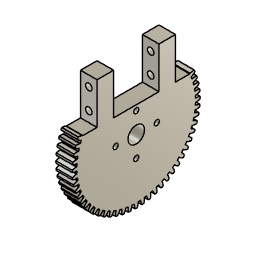
Shaft Arm Joint 0-1 (Autodesk Fusion 360 design; units mm, degrees)
Autodesk Fusion 360 part; units mm, degrees
note: some values were not read from the file. Set by a fixed rule: which sketch regions a step uses.
(part 1 of 59)
sketch "スケッチ1" plane through (0, 0, 0) normal (0, 0, 1) x (1, 0, 0)
  line L0 (4, 19) -> (-4, 19)
  line L1 (-4, 19) -> (-4, -19)
  line L2 (-4, -19) -> (4, -19)
  line L3 (4, -19) -> (4, 19)
  line L4 (4, 19) -> (-4, -19) construction
  line L5 (-4, 19) -> (4, -19) construction
  dimension "d1" = 8
  dimension "d2" = 38
  constraint horizontal L0
  constraint perpendicular L0 L1
  constraint parallel L0 L2
  constraint parallel L1 L3
  constraint coincident L4 origin
  constraint coincident L5 origin
  measures "d1" distance of L1.end L2.end
  measures "d2" distance of L0.end L1.end
extrude "押し出し1" add sketch "スケッチ1" along normal blind 25
sketch "スケッチ4" plane through (4, 0, 0) normal (1, 0, 0) x (0, 1, 0)
  line L0 (-19, 0) -> (19, 0)
  line L1 (19, 0) -> (19, 25)
  line L2 (19, 25) -> (-19, 25)
  line L3 (-19, 25) -> (-19, 0)
  line L4 (0, 25) -> (0, 0)
  circle A0 centre (0, 12.5) radius 12.5
  line L5 (0, 12.5) -> (10, 12.5)
  line L6 (0, 12.5) -> (-10, 12.5)
  line L7 (0, 12.5) -> (0, 22.5)
  line L8 (0, 12.5) -> (0, 2.5)
  line L9 (0, 12.5) -> (7.0711, 5.4289)
  line L10 (0, 12.5) -> (10, 12.5) construction
  line L11 (0, 12.5) -> (7.0711, 19.5711)
  line L12 (0, 12.5) -> (-7.0711, 19.5711)
  line L13 (0, 12.5) -> (-7.0711, 5.4289)
  circle A1 centre (0, 22.5) radius 1.7
  circle A2 centre (7.0711, 19.5711) radius 1.7
  circle A3 centre (10, 12.5) radius 1.7
  circle A4 centre (7.0711, 5.4289) radius 1.7
  circle A5 centre (0, 2.5) radius 1.7
  circle A6 centre (-7.0711, 5.4289) radius 1.7
  circle A7 centre (-10, 12.5) radius 1.7
  circle A8 centre (-7.0711, 19.5711) radius 1.7
  dimension "d11" = 10
  dimension "d12" = 10
  dimension "d13" = 10
  dimension "d14" = 10
  dimension "d15" = 10
  dimension "d16" = 45
  dimension "d17" = 10
  dimension "d18" = 10
  dimension "d19" = 10
  dimension "d20" = 3.4
  dimension "d21" = 3.4
  dimension "d22" = 3.4
  dimension "d23" = 3.4
  dimension "d24" = 3.4
  dimension "d25" = 3.4
  dimension "d26" = 3.4
  dimension "d27" = 3.4
  constraint midpoint L2 L4.start
  constraint coincident L4.end origin
  constraint midpoint L4 A0.centre
  constraint coincident L4.end A0
  constraint coincident A0.centre L5.start
  constraint perpendicular L4 L5
  constraint perpendicular L4 L6
  constraint perpendicular L6 L7
  constraint perpendicular L5 L8
  constraint horizontal L10
  constraint perpendicular L9 L11
  constraint perpendicular L11 L12
  constraint perpendicular L9 L13
  constraint coincident L7.end A1.centre
  constraint coincident L11.end A2.centre
  constraint coincident L5.end L10.end
  constraint coincident L9.end A4.centre
  constraint coincident L8.end A5.centre
  constraint coincident L13.end A6.centre
  constraint coincident L6.end A7.centre
  constraint coincident L12.end A8.centre
  measures "d11" distance of A0.centre L5.end
  measures "d12" distance of A0.centre L6.end
  measures "d13" distance of A0.centre L7.end
  measures "d14" distance of A0.centre L8.end
  measures "d15" distance of A0.centre L9.end
  measures "d16" angle of L9 L10
  measures "d17" distance of A0.centre L11.end
  measures "d18" distance of A0.centre L12.end
  measures "d19" distance of A0.centre L13.end
  measures "d20" diameter of A1
  measures "d21" diameter of A2
  measures "d22" diameter of A3
  measures "d23" diameter of A4
  measures "d24" diameter of A5
  measures "d25" diameter of A6
  measures "d26" diameter of A7
  measures "d27" diameter of A8
extrude "押し出し3" cut sketch "スケッチ4" against normal blind 8 contours L4 L8 A5 | L4 L8 A5 | L4 L7 A1 | L4 L7 A1 | A2 | A3 | A4 | A6 | A7 | A8
sketch "スケッチ6" plane through (0, 0, 25) normal (0, 0, 1) x (-1, 0, 0)
  line L0 (-4, 19) -> (-4, -19)
  line L1 (-4, -19) -> (4, -19)
  line L2 (4, -19) -> (4, 19)
  line L3 (4, 19) -> (-4, 19)
  line L4 (4, -19) -> (-4, -19)
  line L5 (-4, -19) -> (-4, -11)
  line L6 (-4, -11) -> (4, -11)
  line L7 (4, -11) -> (4, -19)
  line L8 (4, 19) -> (-4, 19)
  line L9 (-4, 19) -> (-4, 11)
  line L10 (-4, 11) -> (4, 11)
  line L11 (4, 11) -> (4, 19)
  line L12 (4, -11) -> (-4, -11)
  line L13 (-4, -11) -> (-4, -10)
  line L14 (-4, -10) -> (4, -10)
  line L15 (4, -10) -> (4, -11)
  line L16 (4, 11) -> (-4, 11)
  line L17 (-4, 11) -> (-4, 10)
  line L18 (-4, 10) -> (4, 10)
  line L19 (4, 10) -> (4, 11)
  line L20 (4, -10) -> (-4, -10)
  line L21 (-4, -10) -> (-4, 0)
  line L22 (-4, 0) -> (4, 0)
  line L23 (4, 0) -> (4, -10)
  line L24 (4, 10) -> (-4, 10)
  line L25 (-4, 10) -> (-4, 0)
  line L26 (-4, 0) -> (4, 0)
  line L27 (4, 0) -> (4, 10)
  dimension "d48" = 8
  dimension "d49" = 8
  dimension "d50" = 8
  dimension "d51" = 8
  dimension "d52" = 8
  dimension "d53" = 1
  dimension "d54" = 8
  dimension "d55" = 1
  dimension "d56" = 8
  dimension "d57" = 10
  dimension "d58" = 8
  dimension "d59" = 10
  constraint horizontal L4
  constraint vertical L5
  constraint horizontal L6
  constraint vertical L7
  constraint coincident L1.end L2.start
  constraint horizontal L8
  constraint vertical L9
  constraint horizontal L10
  constraint vertical L11
  constraint coincident L2.end L3.start
  constraint horizontal L12
  constraint vertical L13
  constraint horizontal L14
  constraint vertical L15
  constraint horizontal L16
  constraint vertical L17
  constraint horizontal L18
  constraint vertical L19
  constraint horizontal L20
  constraint vertical L21
  constraint horizontal L22
  constraint vertical L23
  constraint horizontal L24
  constraint vertical L25
  constraint horizontal L26
  constraint vertical L27
  measures "d48" distance of L1.end L0.end
  measures "d49" distance of L1.end L6.end
  measures "d50" distance of L2.end L0.start
  measures "d51" distance of L2.end L10.end
  measures "d52" distance of L6.end L5.end
  measures "d53" distance of L6.end L14.end
  measures "d54" distance of L10.end L9.end
  measures "d55" distance of L10.end L18.end
  measures "d56" distance of L14.end L13.end
  measures "d57" distance of L14.end L22.end
  measures "d58" distance of L18.end L17.end
  measures "d59" distance of L18.end L22.end
extrude "押し出し5" add sketch "スケッチ6" along normal blind 10 contours L0 L2 L3 L8 L9 L10 L11 L16 | L0 L1 L2 L4 L5 L6 L7 L12
sketch "スケッチ7" plane through (4, 0, 0) normal (1, 0, 0) x (0, 1, 0)
  circle A0 centre (-7.0711, 5.4289) radius 1.7
  circle A1 centre (7.0711, 19.5711) radius 1.7
  circle A2 centre (10, 12.5) radius 1.7
  circle A3 centre (0, 2.5) radius 1.7
  circle A4 centre (-10, 12.5) radius 1.7
  circle A5 centre (0, 22.5) radius 1.7
  circle A6 centre (-7.0711, 19.5711) radius 1.7
  circle A7 centre (7.0711, 5.4289) radius 1.7
  line L0 (-19, 0) -> (19, 0)
  line L1 (19, 0) -> (19, 35)
  line L2 (19, 35) -> (11, 35)
  line L3 (11, 35) -> (11, 25)
  line L4 (11, 25) -> (-11, 25)
  line L5 (-11, 25) -> (-11, 35)
  line L6 (-11, 35) -> (-19, 35)
  line L7 (-19, 35) -> (-19, 0)
  circle A8 centre (0, 12.5) radius 12.5
  line L8 (-11, 25) -> (-19, 25)
  line L9 (11, 25) -> (19, 25)
  line L10 (19, 25) -> (11.479, 7.552)
  line L11 (-19, 25) -> (-11.479, 7.552)
  constraint tangent L4 A8
  constraint coincident L4.end L5.start
  constraint coincident L7 L8.end
  constraint perpendicular L7 L8
  constraint coincident L3.end L4.start
  constraint coincident L1 L9.end
  constraint perpendicular L1 L9
  constraint coincident A8 L10.end
  constraint tangent A8 L10
  constraint coincident A8 L11.end
  constraint tangent A8 L11
extrude "押し出し6" cut sketch "スケッチ7" against normal blind 8 contours L0 L7 A8 L11 | L0 L1 A8 L10
sketch "スケッチ8" plane through (4, 0, 0) normal (1, 0, 0) x (0, 1, 0)
  circle A0 centre (7.0711, 5.4289) radius 1.7
  circle A1 centre (-7.0711, 19.5711) radius 1.7
  circle A2 centre (0, 22.5) radius 1.7
  circle A3 centre (-10, 12.5) radius 1.7
  circle A4 centre (0, 2.5) radius 1.7
  circle A5 centre (10, 12.5) radius 1.7
  circle A6 centre (7.0711, 19.5711) radius 1.7
  circle A7 centre (-7.0711, 5.4289) radius 1.7
  line L0 (-19, 25) -> (-11.479, 7.552)
  arc A8 (-11.479, 7.552) -> (11.479, 7.552) centre (0, 12.5) ccw
  line L1 (11.479, 7.552) -> (19, 25)
  line L2 (19, 25) -> (19, 35)
  line L3 (19, 35) -> (11, 35)
  line L4 (11, 35) -> (11, 25)
  line L5 (11, 25) -> (-11, 25)
  line L6 (-11, 25) -> (-11, 35)
  line L7 (-11, 35) -> (-19, 35)
  line L8 (-19, 35) -> (-19, 25)
  circle A9 centre (0, 12.5) radius 13.7
  line L9 (19, 25) -> (12.9047, 7.9001)
  line L10 (-19, 25) -> (-12.9047, 7.9001)
  dimension "d64" = 27.4
  constraint concentric A8 A9
  constraint coincident L1.end L2.start
  constraint coincident A9 L9.end
  constraint tangent A9 L9
  constraint coincident L0.start L8.end
  constraint coincident A9 L10.end
  constraint tangent A9 L10
  measures "d64" diameter of A9
extrude "押し出し7" add sketch "スケッチ8" against normal blind 8 contours L0 A9 L10 | L0 A8 L1 A9 | L1 A9 L9
sketch "スケッチ9" plane through (4, 0, 0) normal (1, 0, 0) x (0, 1, 0)
  circle A0 centre (7.0711, 5.4289) radius 1.7
  circle A1 centre (-7.0711, 19.5711) radius 1.7
  circle A2 centre (0, 22.5) radius 1.7
  circle A3 centre (-10, 12.5) radius 1.7
  circle A4 centre (0, 2.5) radius 1.7
  circle A5 centre (10, 12.5) radius 1.7
  circle A6 centre (7.0711, 19.5711) radius 1.7
  circle A7 centre (-7.0711, 5.4289) radius 1.7
  line L0 (-19, 25) -> (-12.9047, 7.9001)
  arc A8 (-12.9047, 7.9001) -> (12.9047, 7.9001) centre (0, 12.5) ccw
  line L1 (12.9047, 7.9001) -> (19, 25)
  line L2 (19, 25) -> (19, 35)
  line L3 (19, 35) -> (11, 35)
  line L4 (11, 35) -> (11, 25)
  line L5 (11, 25) -> (-11, 25)
  line L6 (-11, 25) -> (-11, 35)
  line L7 (-11, 35) -> (-19, 35)
  line L8 (-19, 35) -> (-19, 25)
  line L9 (0, 12.5) -> (0, 12.2)
  line L10 (0, 12.5) -> (0, 12.8)
  line L11 (3, 12.2) -> (-3, 12.2)
  line L12 (-3, 12.2) -> (-3, 12.8)
  line L13 (-3, 12.8) -> (3, 12.8)
  line L14 (3, 12.8) -> (3, 12.2)
  line L15 (3, 12.2) -> (-3, 12.8) construction
  line L16 (-3, 12.2) -> (3, 12.8) construction
  line L17 (0, 12.8) -> (0, 15.3)
  line L18 (0, 12.2) -> (0, 9.7)
  circle A9 centre (0, 12.8) radius 3
  circle A10 centre (0, 12.2) radius 3
  point P0 (0, 12.5)
  dimension "d69" = 0.3
  dimension "d70" = 0.3
  dimension "d71" = 6
  dimension "d72" = 2.5
  dimension "d73" = 2.5
  constraint coincident P0 A8.centre
  constraint vertical L9
  constraint parallel L9 L10
  constraint horizontal L11
  constraint perpendicular L11 L12
  constraint parallel L11 L13
  constraint parallel L12 L14
  constraint coincident L15 P0
  constraint coincident L16 P0
  constraint perpendicular L13 L17
  constraint perpendicular L11 L18
  constraint coincident L10.end L17.start
  constraint coincident L13.end A9
  constraint coincident L11.start A10
  measures "d69" distance of P0 L9.end
  measures "d70" distance of P0 L10.end
  measures "d71" distance of L12.end L13.end
  measures "d72" distance of L10.end L17.end
  measures "d73" distance of L9.end L18.end
extrude "押し出し8" cut sketch "スケッチ9" against normal blind 8 contours L11 L18 A9 | L11 L18 A9 | L13 L17 A10 | L13 L17 A10 | L11 A9 A10 | L13 A9 A10 picked at (0, 9.4056) picked at (0, 15.5944)
sketch "スケッチ10" plane through (4, 0, 0) normal (1, 0, 0) x (0, 1, 0)
  line L0 (3, 12.8) -> (-3, 12.8)
  arc A0 (3, 12.8) -> (-3, 12.8) centre (0, 12.8) ccw
  arc A1 (-3, 12.2) -> (3, 12.2) centre (0, 12.2) ccw
  line L1 (-3, 12.2) -> (3, 12.2)
  circle A2 centre (7.0711, 5.4289) radius 1.7
  circle A3 centre (-7.0711, 19.5711) radius 1.7
  circle A4 centre (0, 22.5) radius 1.7
  circle A5 centre (-10, 12.5) radius 1.7
  circle A6 centre (0, 2.5) radius 1.7
  circle A7 centre (10, 12.5) radius 1.7
  circle A8 centre (7.0711, 19.5711) radius 1.7
  circle A9 centre (-7.0711, 5.4289) radius 1.7
  line L2 (-19, 25) -> (-12.9047, 7.9001)
  arc A10 (-12.9047, 7.9001) -> (12.9047, 7.9001) centre (0, 12.5) ccw
  line L3 (12.9047, 7.9001) -> (19, 25)
  line L4 (19, 25) -> (19, 35)
  line L5 (19, 35) -> (11, 35)
  line L6 (11, 35) -> (11, 25)
  line L7 (11, 25) -> (-11, 25)
  line L8 (-11, 25) -> (-11, 35)
  line L9 (-11, 35) -> (-19, 35)
  line L10 (-19, 35) -> (-19, 25)
  line L11 (-19, 25) -> (-20, 25)
  line L12 (19, 25) -> (20, 25)
  line L13 (-20, 25) -> (-12.6588, 7.2612)
  line L14 (20, 25) -> (12.6588, 7.2612)
  dimension "d76" = 1
  dimension "d77" = 1
  constraint coincident L2.start L10.end
  constraint perpendicular L10 L11
  constraint coincident L3.end L4.start
  constraint perpendicular L4 L12
  constraint coincident A10 L13.end
  constraint tangent A10 L13
  constraint coincident A10 L14.end
  constraint tangent A10 L14
  measures "d76" distance of L2.start L11.end
  measures "d77" distance of L3.end L12.end
extrude "押し出し9" add sketch "スケッチ10" against normal blind 8 contours L2 A10 L11 L13 | A10 L3 L12 L14
cylinder "円柱プリミティブ1" cut diameter 3.4 height -38 placed x (1, 0, 0) y (0, 0, 1) z (0, -1, 0) at (0, -19, 30)
sketch "スケッチ15" plane through (4, 0, 0) normal (1, 0, 0) x (0, 1, 0)
  line L0 (3, 12.8) -> (-3, 12.8)
  arc A0 (3, 12.8) -> (-3, 12.8) centre (0, 12.8) ccw
  arc A1 (-3, 12.2) -> (3, 12.2) centre (0, 12.2) ccw
  line L1 (-3, 12.2) -> (3, 12.2)
  circle A2 centre (7.0711, 5.4289) radius 1.7
  circle A3 centre (-7.0711, 19.5711) radius 1.7
  circle A4 centre (0, 22.5) radius 1.7
  circle A5 centre (-10, 12.5) radius 1.7
  circle A6 centre (0, 2.5) radius 1.7
  circle A7 centre (10, 12.5) radius 1.7
  circle A8 centre (7.0711, 19.5711) radius 1.7
  circle A9 centre (-7.0711, 5.4289) radius 1.7
  arc A10 (-12.6588, 7.2612) -> (12.6588, 7.2612) centre (0, 12.5) ccw
  line L2 (12.6588, 7.2612) -> (20, 25)
  line L3 (20, 25) -> (19, 25)
  line L4 (19, 25) -> (19, 35)
  line L5 (19, 35) -> (11, 35)
  line L6 (11, 35) -> (11, 25)
  line L7 (11, 25) -> (-11, 25)
  line L8 (-11, 25) -> (-11, 35)
  line L9 (-11, 35) -> (-19, 35)
  line L10 (-19, 35) -> (-19, 25)
  line L11 (-19, 25) -> (-20, 25)
  line L12 (-20, 25) -> (-12.6588, 7.2612)
  line L13 (22.1904, -6.2406) -> (22.1898, -6.2401)
  line L14 (26.6221, 23.3547) -> (26.8948, 23.4659)
  line L15 (25.3417, 26.078) -> (25.6012, 26.2171)
  line L16 (17.8091, -10.4448) -> (17.8086, -10.4441)
  line L17 (17.8086, -10.4441) -> (17.6281, -10.2115)
  spline S0 degree 5 poles (27.8945, 20.5948) (27.8946, 20.5948) (27.8948, 20.5948) (27.8951, 20.5949) (27.8956, 20.5951) (27.8963, 20.5953) (27.8971, 20.5956) (27.898, 20.5958) (27.8991, 20.5962) (27.9002, 20.5965) (27.9015, 20.5969) (27.9028, 20.5973) (27.9043, 20.5978) (27.9058, 20.5983) (27.9075, 20.5988) (27.9092, 20.5994) (27.9111, 20.6) (27.913, 20.6007) (27.915, 20.6013) (27.9172, 20.602) (27.9194, 20.6028) (27.9217, 20.6036) (27.9241, 20.6044) (27.9265, 20.6052) (27.9291, 20.6061) (27.9318, 20.607) (27.9345, 20.608) (27.9373, 20.609) (27.9402, 20.61) (27.9432, 20.6111) (27.9462, 20.6121) (27.9494, 20.6133) (27.9526, 20.6144) (27.9559, 20.6156) (27.9593, 20.6169) (27.9627, 20.6181) (27.9662, 20.6194) (27.9698, 20.6208) (27.9735, 20.6222) (27.9772, 20.6236) (27.9811, 20.625) (27.9849, 20.6265) (27.9889, 20.628) (27.9929, 20.6295) (27.997, 20.6311) (28.0012, 20.6327) (28.0054, 20.6344) (28.0097, 20.6361) (28.0141, 20.6378) (28.0185, 20.6395) (28.023, 20.6413) (28.0276, 20.6432) (28.0322, 20.645) (28.0369, 20.6469) (28.0416, 20.6488) (28.0464, 20.6508) (28.0513, 20.6528) (28.0562, 20.6548) (28.0612, 20.6569) (28.0663, 20.659) (28.0714, 20.6611) (28.0765, 20.6633) (28.0818, 20.6655) (28.087, 20.6677) (28.0924, 20.67) (28.0978, 20.6723) (28.1032, 20.6747) (28.1087, 20.677) (28.1143, 20.6795) (28.1199, 20.6819) (28.1256, 20.6844) (28.1313, 20.6869) (28.1371, 20.6895) (28.1429, 20.692) (28.1488, 20.6947) (28.1547, 20.6973) (28.1607, 20.7) (28.1667, 20.7027) (28.1728, 20.7055) (28.179, 20.7083) (28.1851, 20.7111) (28.1914, 20.714) (28.1977, 20.7169) (28.204, 20.7198) (28.2104, 20.7227) (28.2168, 20.7257) (28.2233, 20.7288) (28.2298, 20.7318) (28.2363, 20.7349) (28.2429, 20.7381) (28.2496, 20.7412) (28.2563, 20.7445) (28.263, 20.7477) (28.2698, 20.751) (28.2767, 20.7543) (28.2835, 20.7576) (28.2905, 20.761) (28.2974, 20.7644) (28.3044, 20.7678) (28.3115, 20.7713) (28.3186, 20.7748) (28.3257, 20.7784) (28.3329, 20.782) (28.3401, 20.7856) (28.3473, 20.7892) (28.3546, 20.7929) (28.3619, 20.7966) (28.3693, 20.8004) (28.3767, 20.8042) (28.3842, 20.808) (28.3917, 20.8118) (28.3992, 20.8157) (28.4068, 20.8196) (28.4144, 20.8236) (28.422, 20.8276) (28.4297, 20.8316) (28.4374, 20.8357) (28.4452, 20.8398) (28.4529, 20.8439) (28.4608, 20.848) (28.4686, 20.8522) (28.4765, 20.8565) (28.4845, 20.8607) (28.4924, 20.865) (28.5004, 20.8693) (28.5085, 20.8737) (28.5165, 20.8781) (28.5246, 20.8825) (28.5328, 20.887) (28.5409, 20.8915) (28.5491, 20.896) (28.5574, 20.9006) (28.5657, 20.9052) (28.574, 20.9098) (28.5823, 20.9145) (28.5907, 20.9192) (28.5991, 20.9239) (28.6075, 20.9287) (28.616, 20.9335) (28.6244, 20.9384) (28.633, 20.9432) (28.6415, 20.9481) (28.6501, 20.9531) (28.6587, 20.958) (28.6674, 20.963) (28.676, 20.9681) (28.6847, 20.9732) (28.6935, 20.9783) (28.7022, 20.9834) (28.711, 20.9886) (28.7199, 20.9938) (28.7287, 20.999) (28.7376, 21.0043) (28.7465, 21.0096) (28.7554, 21.015) (28.7644, 21.0203) (28.7734, 21.0257) (28.7824, 21.0312) (28.7914, 21.0367) (28.8005, 21.0422) (28.8096, 21.0477) (28.8187, 21.0533) (28.8279, 21.0589) (28.837, 21.0645) (28.8462, 21.0702) (28.8555, 21.0759) (28.8647, 21.0817) (28.874, 21.0874) (28.8833, 21.0932) (28.8926, 21.0991) (28.902, 21.105) (28.9113, 21.1109) (28.9207, 21.1168) (28.9302, 21.1228) (28.9396, 21.1288) (28.9491, 21.1348) (28.9586, 21.1409) (28.9681, 21.147) (28.9776, 21.1532) (28.9872, 21.1593) (28.9968, 21.1656) (29.0064, 21.1718) (29.016, 21.1781) (29.0257, 21.1844) (29.0354, 21.1907) (29.0451, 21.1971) (29.0548, 21.2035) (29.0646, 21.2099) (29.0743, 21.2164) (29.0841, 21.2229) (29.0939, 21.2295) (29.1037, 21.236) (29.1136, 21.2426) (29.1235, 21.2493) (29.1334, 21.2559) (29.1433, 21.2626) (29.1532, 21.2694) (29.1632, 21.2762) (29.1731, 21.283) (29.1831, 21.2898) (29.1932, 21.2967) (29.2032, 21.3036) (29.2132, 21.3105) (29.2233, 21.3175) (29.2334, 21.3245) (29.2435, 21.3315) (29.2537, 21.3386) (29.2638, 21.3457) (29.274, 21.3528) (29.2842, 21.36) (29.2944, 21.3671) (29.3046, 21.3744) (29.3148, 21.3816) (29.3251, 21.3889) (29.3354, 21.3963) (29.3457, 21.4036) (29.356, 21.411) (29.3663, 21.4184) (29.3766, 21.4259) (29.387, 21.4334) (29.3974, 21.4409) (29.4078, 21.4485) (29.4182, 21.456) (29.4286, 21.4637) (29.4391, 21.4713) (29.4495, 21.479) (29.46, 21.4867) (29.4705, 21.4945) (29.481, 21.5022) (29.4915, 21.5101) (29.5021, 21.5179) (29.5127, 21.5258) (29.5232, 21.5337) (29.5338, 21.5416) (29.5444, 21.5496) (29.555, 21.5576) (29.5657, 21.5657) (29.5763, 21.5737) (29.587, 21.5818) (29.5977, 21.59) (29.6084, 21.5981) (29.6169, 21.6047) (29.6234, 21.6096) (29.6276, 21.6129) (29.6298, 21.6146) knots 0 0 0 0 0 0 0.00416667 0.00833333 0.0125 0.01666667 0.02083333 0.025 0.02916667 0.03333333 0.0375 0.04166667 0.04583333 0.05 0.05416667 0.05833333 0.0625 0.06666667 0.07083333 0.075 0.07916667 0.08333333 0.0875 0.09166667 0.09583333 0.1 0.10416667 0.10833333 0.1125 0.11666667 0.12083333 0.125 0.12916667 0.13333333 0.1375 0.14166667 0.14583333 0.15 0.15416667 0.15833333 0.1625 0.16666667 0.17083333 0.175 0.17916667 0.18333333 0.1875 0.19166667 0.19583333 0.2 0.20416667 0.20833333 0.2125 0.21666667 0.22083333 0.225 0.22916667 0.23333333 0.2375 0.24166667 0.24583333 0.25 0.25416667 0.25833333 0.2625 0.26666667 0.27083333 0.275 0.27916667 0.28333333 0.2875 0.29166667 0.29583333 0.3 0.30416667 0.30833333 0.3125 0.31666667 0.32083333 0.325 0.32916667 0.33333333 0.3375 0.34166667 0.34583333 0.35 0.35416667 0.35833333 0.3625 0.36666667 0.37083333 0.375 0.37916667 0.38333333 0.3875 0.39166667 0.39583333 0.4 0.40416667 0.40833333 0.4125 0.41666667 0.42083333 0.425 0.42916667 0.43333333 0.4375 0.44166667 0.44583333 0.45 0.45416667 0.45833333 0.4625 0.46666667 0.47083333 0.475 0.47916667 0.48333333 0.4875 0.49166667 0.49583333 0.5 0.50416667 0.50833333 0.5125 0.51666667 0.52083333 0.525 0.52916667 0.53333333 0.5375 0.54166667 0.54583333 0.55 0.55416667 0.55833333 0.5625 0.56666667 0.57083333 0.575 0.57916667 0.58333333 0.5875 0.59166667 0.59583333 0.6 0.60416667 0.60833333 0.6125 0.61666667 0.62083333 0.625 0.62916667 0.63333333 0.6375 0.64166667 0.64583333 0.65 0.65416667 0.65833333 0.6625 0.66666667 0.67083333 0.675 0.67916667 0.68333333 0.6875 0.69166667 0.69583333 0.7 0.70416667 0.70833333 0.7125 0.71666667 0.72083333 0.725 0.72916667 0.73333333 0.7375 0.74166667 0.74583333 0.75 0.75416667 0.75833333 0.7625 0.76666667 0.77083333 0.775 0.77916667 0.78333333 0.7875 0.79166667 0.79583333 0.8 0.80416667 0.80833333 0.8125 0.81666667 0.82083333 0.825 0.82916667 0.83333333 0.8375 0.84166667 0.84583333 0.85 0.85416667 0.85833333 0.8625 0.86666667 0.87083333 0.875 0.87916667 0.88333333 0.8875 0.89166667 0.89583333 0.9 0.90416667 0.90833333 0.9125 0.91666667 0.92083333 0.925 0.92916667 0.93333333 0.9375 0.94166667 0.94583333 0.95 0.95416667 0.95833333 0.9625 0.96666667 0.97083333 0.975 0.97916667 0.98333333 0.9875 0.99166667 0.99583333 1 1 1 1 1 1
  spline S1 degree 5 poles (3.7249, -18.2754) (3.7256, -18.2728) (3.7268, -18.2675) (3.7287, -18.2596) (3.7312, -18.2491) (3.7343, -18.236) (3.7374, -18.223) (3.7405, -18.2099) (3.7435, -18.1969) (3.7466, -18.1839) (3.7496, -18.171) (3.7525, -18.158) (3.7555, -18.1451) (3.7584, -18.1323) (3.7613, -18.1194) (3.7642, -18.1066) (3.767, -18.0938) (3.7699, -18.081) (3.7727, -18.0683) (3.7755, -18.0556) (3.7782, -18.0429) (3.781, -18.0302) (3.7837, -18.0176) (3.7864, -18.005) (3.7891, -17.9924) (3.7917, -17.9799) (3.7943, -17.9674) (3.797, -17.9549) (3.7995, -17.9424) (3.8021, -17.93) (3.8046, -17.9176) (3.8071, -17.9053) (3.8096, -17.8929) (3.8121, -17.8806) (3.8145, -17.8683) (3.817, -17.8561) (3.8194, -17.8439) (3.8217, -17.8317) (3.8241, -17.8195) (3.8264, -17.8074) (3.8288, -17.7953) (3.831, -17.7832) (3.8333, -17.7712) (3.8356, -17.7592) (3.8378, -17.7472) (3.84, -17.7353) (3.8422, -17.7233) (3.8443, -17.7115) (3.8464, -17.6996) (3.8486, -17.6878) (3.8507, -17.676) (3.8527, -17.6643) (3.8548, -17.6525) (3.8568, -17.6409) (3.8588, -17.6292) (3.8608, -17.6176) (3.8628, -17.606) (3.8647, -17.5944) (3.8666, -17.5829) (3.8685, -17.5714) (3.8704, -17.56) (3.8722, -17.5486) (3.8741, -17.5372) (3.8759, -17.5258) (3.8777, -17.5145) (3.8795, -17.5032) (3.8812, -17.492) (3.8829, -17.4807) (3.8846, -17.4696) (3.8863, -17.4584) (3.888, -17.4473) (3.8896, -17.4362) (3.8913, -17.4252) (3.8929, -17.4142) (3.8945, -17.4032) (3.896, -17.3923) (3.8976, -17.3814) (3.8991, -17.3705) (3.9006, -17.3597) (3.9021, -17.3489) (3.9035, -17.3382) (3.905, -17.3274) (3.9064, -17.3168) (3.9078, -17.3061) (3.9092, -17.2955) (3.9106, -17.285) (3.9119, -17.2744) (3.9132, -17.264) (3.9145, -17.2535) (3.9158, -17.2431) (3.9171, -17.2327) (3.9183, -17.2224) (3.9196, -17.2121) (3.9208, -17.2018) (3.922, -17.1916) (3.9231, -17.1814) (3.9243, -17.1713) (3.9254, -17.1612) (3.9265, -17.1512) (3.9276, -17.1411) (3.9287, -17.1312) (3.9297, -17.1212) (3.9308, -17.1113) (3.9318, -17.1015) (3.9328, -17.0917) (3.9338, -17.0819) (3.9348, -17.0722) (3.9357, -17.0625) (3.9366, -17.0529) (3.9375, -17.0433) (3.9384, -17.0337) (3.9393, -17.0242) (3.9402, -17.0147) (3.941, -17.0053) (3.9418, -16.9959) (3.9426, -16.9866) (3.9434, -16.9773) (3.9442, -16.968) (3.9449, -16.9588) (3.9457, -16.9497) (3.9464, -16.9406) (3.9471, -16.9315) (3.9478, -16.9225) (3.9484, -16.9135) (3.9491, -16.9045) (3.9497, -16.8957) (3.9503, -16.8868) (3.9509, -16.878) (3.9515, -16.8693) (3.9521, -16.8606) (3.9526, -16.8519) (3.9532, -16.8433) (3.9537, -16.8348) (3.9542, -16.8263) (3.9547, -16.8178) (3.9552, -16.8094) (3.9556, -16.801) (3.9561, -16.7927) (3.9565, -16.7845) (3.9569, -16.7763) (3.9573, -16.7681) (3.9577, -16.76) (3.9581, -16.7519) (3.9584, -16.7439) (3.9588, -16.736) (3.9591, -16.7281) (3.9594, -16.7202) (3.9597, -16.7124) (3.96, -16.7047) (3.9603, -16.697) (3.9605, -16.6893) (3.9607, -16.6817) (3.961, -16.6742) (3.9612, -16.6667) (3.9614, -16.6593) (3.9616, -16.6519) (3.9618, -16.6446) (3.9619, -16.6374) (3.9621, -16.6302) (3.9622, -16.623) (3.9623, -16.6159) (3.9625, -16.6089) (3.9626, -16.6019) (3.9626, -16.595) (3.9627, -16.5882) (3.9628, -16.5814) (3.9628, -16.5746) (3.9629, -16.568) (3.9629, -16.5613) (3.9629, -16.5548) (3.963, -16.5483) (3.963, -16.5418) (3.9629, -16.5355) (3.9629, -16.5291) (3.9629, -16.5229) (3.9629, -16.5167) (3.9628, -16.5106) (3.9627, -16.5045) (3.9627, -16.4985) (3.9626, -16.4926) (3.9625, -16.4867) (3.9624, -16.4809) (3.9623, -16.4752) (3.9622, -16.4695) (3.9621, -16.4639) (3.962, -16.4584) (3.9618, -16.4529) (3.9617, -16.4475) (3.9615, -16.4422) (3.9614, -16.4369) (3.9612, -16.4317) (3.961, -16.4266) (3.9609, -16.4215) (3.9607, -16.4166) (3.9605, -16.4117) (3.9603, -16.4068) (3.9601, -16.4021) (3.9599, -16.3974) (3.9597, -16.3928) (3.9595, -16.3882) (3.9593, -16.3838) (3.959, -16.3794) (3.9588, -16.3751) (3.9586, -16.3709) (3.9584, -16.3667) (3.9581, -16.3626) (3.9579, -16.3586) (3.9577, -16.3547) (3.9574, -16.3509) (3.9572, -16.3472) (3.9569, -16.3435) (3.9567, -16.3399) (3.9564, -16.3364) (3.9562, -16.333) (3.9559, -16.3297) (3.9557, -16.3264) (3.9555, -16.3233) (3.9552, -16.3202) (3.955, -16.3172) (3.9547, -16.3144) (3.9545, -16.3116) (3.9543, -16.3089) (3.954, -16.3063) (3.9538, -16.3037) (3.9536, -16.3013) (3.9534, -16.299) (3.9531, -16.2968) (3.9529, -16.2946) (3.9527, -16.2926) (3.9525, -16.2907) (3.9523, -16.2889) (3.9522, -16.2871) (3.952, -16.2855) (3.9518, -16.284) (3.9517, -16.2826) (3.9515, -16.2813) (3.9514, -16.2801) (3.9512, -16.279) (3.9511, -16.278) (3.951, -16.2772) (3.9509, -16.2764) (3.9509, -16.2759) (3.9508, -16.2756) (3.9508, -16.2754) (3.9508, -16.2753) knots -1 -1 -1 -1 -1 -1 -0.99583333 -0.99166667 -0.9875 -0.98333333 -0.97916667 -0.975 -0.97083333 -0.96666667 -0.9625 -0.95833333 -0.95416667 -0.95 -0.94583333 -0.94166667 -0.9375 -0.93333333 -0.92916667 -0.925 -0.92083333 -0.91666667 -0.9125 -0.90833333 -0.90416667 -0.9 -0.89583333 -0.89166667 -0.8875 -0.88333333 -0.87916667 -0.875 -0.87083333 -0.86666667 -0.8625 -0.85833333 -0.85416667 -0.85 -0.84583333 -0.84166667 -0.8375 -0.83333333 -0.82916667 -0.825 -0.82083333 -0.81666667 -0.8125 -0.80833333 -0.80416667 -0.8 -0.79583333 -0.79166667 -0.7875 -0.78333333 -0.77916667 -0.775 -0.77083333 -0.76666667 -0.7625 -0.75833333 -0.75416667 -0.75 -0.74583333 -0.74166667 -0.7375 -0.73333333 -0.72916667 -0.725 -0.72083333 -0.71666667 -0.7125 -0.70833333 -0.70416667 -0.7 -0.69583333 -0.69166667 -0.6875 -0.68333333 -0.67916667 -0.675 -0.67083333 -0.66666667 -0.6625 -0.65833333 -0.65416667 -0.65 -0.64583333 -0.64166667 -0.6375 -0.63333333 -0.62916667 -0.625 -0.62083333 -0.61666667 -0.6125 -0.60833333 -0.60416667 -0.6 -0.59583333 -0.59166667 -0.5875 -0.58333333 -0.57916667 -0.575 -0.57083333 -0.56666667 -0.5625 -0.55833333 -0.55416667 -0.55 -0.54583333 -0.54166667 -0.5375 -0.53333333 -0.52916667 -0.525 -0.52083333 -0.51666667 -0.5125 -0.50833333 -0.50416667 -0.5 -0.49583333 -0.49166667 -0.4875 -0.48333333 -0.47916667 -0.475 -0.47083333 -0.46666667 -0.4625 -0.45833333 -0.45416667 -0.45 -0.44583333 -0.44166667 -0.4375 -0.43333333 -0.42916667 -0.425 -0.42083333 -0.41666667 -0.4125 -0.40833333 -0.40416667 -0.4 -0.39583333 -0.39166667 -0.3875 -0.38333333 -0.37916667 -0.375 -0.37083333 -0.36666667 -0.3625 -0.35833333 -0.35416667 -0.35 -0.34583333 -0.34166667 -0.3375 -0.33333333 -0.32916667 -0.325 -0.32083333 -0.31666667 -0.3125 -0.30833333 -0.30416667 -0.3 -0.29583333 -0.29166667 -0.2875 -0.28333333 -0.27916667 -0.275 -0.27083333 -0.26666667 -0.2625 -0.25833333 -0.25416667 -0.25 -0.24583333 -0.24166667 -0.2375 -0.23333333 -0.22916667 -0.225 -0.22083333 -0.21666667 -0.2125 -0.20833333 -0.20416667 -0.2 -0.19583333 -0.19166667 -0.1875 -0.18333333 -0.17916667 -0.175 -0.17083333 -0.16666667 -0.1625 -0.15833333 -0.15416667 -0.15 -0.14583333 -0.14166667 -0.1375 -0.13333333 -0.12916667 -0.125 -0.12083333 -0.11666667 -0.1125 -0.10833333 -0.10416667 -0.1 -0.09583333 -0.09166667 -0.0875 -0.08333333 -0.07916667 -0.075 -0.07083333 -0.06666667 -0.0625 -0.05833333 -0.05416667 -0.05 -0.04583333 -0.04166667 -0.0375 -0.03333333 -0.02916667 -0.025 -0.02083333 -0.01666667 -0.0125 -0.00833333 -0.00416667 0 0 0 0 0 0
  line L18 (24.6799, 27.8128) -> (24.4297, 27.6575)
  arc A11 (29.6298, 21.6146) -> (29.3284, 22.5421) centre (0, 12.5) ccw
  line L19 (26.8948, 23.4659) -> (26.8955, 23.4662)
  line L20 (24.0278, -3.8184) -> (24.0271, -3.818)
  line L21 (24.0271, -3.818) -> (23.7836, -3.6526)
  line L22 (24.6806, 27.8132) -> (24.6799, 27.8128)
  arc A12 (30.4202, 18.4675) -> (30.2174, 19.4214) centre (0, 12.5) ccw
  arc A13 (27.918, 19.3665) -> (27.6109, 20.5125) centre (0, 12.5) ccw
  spline S2 degree 5 poles (-5.9675, -17.9202) (-5.9661, -17.9179) (-5.9633, -17.9133) (-5.959, -17.9064) (-5.9534, -17.8972) (-5.9464, -17.8857) (-5.9394, -17.8742) (-5.9325, -17.8628) (-5.9255, -17.8513) (-5.9187, -17.8399) (-5.9118, -17.8285) (-5.905, -17.8171) (-5.8982, -17.8058) (-5.8914, -17.7944) (-5.8847, -17.7831) (-5.878, -17.7718) (-5.8713, -17.7605) (-5.8647, -17.7492) (-5.8581, -17.738) (-5.8515, -17.7268) (-5.8449, -17.7156) (-5.8384, -17.7044) (-5.8319, -17.6932) (-5.8255, -17.6821) (-5.8191, -17.6709) (-5.8127, -17.6598) (-5.8063, -17.6487) (-5.8, -17.6377) (-5.7937, -17.6266) (-5.7874, -17.6156) (-5.7811, -17.6046) (-5.7749, -17.5936) (-5.7688, -17.5826) (-5.7626, -17.5717) (-5.7565, -17.5608) (-5.7504, -17.5499) (-5.7443, -17.539) (-5.7383, -17.5281) (-5.7323, -17.5173) (-5.7263, -17.5065) (-5.7204, -17.4957) (-5.7145, -17.4849) (-5.7086, -17.4742) (-5.7028, -17.4634) (-5.697, -17.4527) (-5.6912, -17.4421) (-5.6854, -17.4314) (-5.6797, -17.4208) (-5.674, -17.4102) (-5.6683, -17.3996) (-5.6627, -17.389) (-5.6571, -17.3785) (-5.6515, -17.368) (-5.646, -17.3575) (-5.6405, -17.347) (-5.635, -17.3366) (-5.6296, -17.3262) (-5.6242, -17.3158) (-5.6188, -17.3054) (-5.6134, -17.2951) (-5.6081, -17.2847) (-5.6028, -17.2745) (-5.5975, -17.2642) (-5.5923, -17.254) (-5.5871, -17.2437) (-5.5819, -17.2336) (-5.5768, -17.2234) (-5.5717, -17.2133) (-5.5666, -17.2032) (-5.5615, -17.1931) (-5.5565, -17.183) (-5.5515, -17.173) (-5.5466, -17.163) (-5.5416, -17.153) (-5.5367, -17.1431) (-5.5319, -17.1332) (-5.527, -17.1233) (-5.5222, -17.1134) (-5.5175, -17.1036) (-5.5127, -17.0938) (-5.508, -17.084) (-5.5033, -17.0743) (-5.4987, -17.0646) (-5.494, -17.0549) (-5.4895, -17.0452) (-5.4849, -17.0356) (-5.4804, -17.026) (-5.4759, -17.0165) (-5.4714, -17.0069) (-5.467, -16.9974) (-5.4625, -16.9879) (-5.4582, -16.9785) (-5.4538, -16.9691) (-5.4495, -16.9597) (-5.4452, -16.9504) (-5.441, -16.941) (-5.4367, -16.9318) (-5.4325, -16.9225) (-5.4284, -16.9133) (-5.4242, -16.9041) (-5.4201, -16.895) (-5.4161, -16.8858) (-5.412, -16.8767) (-5.408, -16.8677) (-5.404, -16.8587) (-5.4001, -16.8497) (-5.3961, -16.8407) (-5.3922, -16.8318) (-5.3884, -16.8229) (-5.3846, -16.8141) (-5.3807, -16.8053) (-5.377, -16.7965) (-5.3732, -16.7878) (-5.3695, -16.779) (-5.3658, -16.7704) (-5.3622, -16.7617) (-5.3586, -16.7531) (-5.355, -16.7446) (-5.3514, -16.7361) (-5.3479, -16.7276) (-5.3444, -16.7191) (-5.3409, -16.7107) (-5.3375, -16.7023) (-5.3341, -16.694) (-5.3307, -16.6857) (-5.3273, -16.6775) (-5.324, -16.6692) (-5.3207, -16.6611) (-5.3175, -16.6529) (-5.3143, -16.6448) (-5.3111, -16.6368) (-5.3079, -16.6288) (-5.3047, -16.6208) (-5.3016, -16.6129) (-5.2986, -16.605) (-5.2955, -16.5971) (-5.2925, -16.5893) (-5.2895, -16.5815) (-5.2865, -16.5738) (-5.2836, -16.5661) (-5.2807, -16.5585) (-5.2778, -16.5509) (-5.275, -16.5433) (-5.2722, -16.5358) (-5.2694, -16.5284) (-5.2666, -16.521) (-5.2639, -16.5136) (-5.2612, -16.5063) (-5.2586, -16.499) (-5.2559, -16.4918) (-5.2533, -16.4846) (-5.2508, -16.4774) (-5.2482, -16.4703) (-5.2457, -16.4633) (-5.2432, -16.4563) (-5.2408, -16.4493) (-5.2383, -16.4424) (-5.2359, -16.4356) (-5.2336, -16.4288) (-5.2312, -16.422) (-5.2289, -16.4153) (-5.2266, -16.4087) (-5.2244, -16.4021) (-5.2222, -16.3955) (-5.22, -16.389) (-5.2178, -16.3826) (-5.2157, -16.3762) (-5.2136, -16.3699) (-5.2115, -16.3636) (-5.2094, -16.3573) (-5.2074, -16.3512) (-5.2054, -16.3451) (-5.2035, -16.339) (-5.2015, -16.333) (-5.1996, -16.327) (-5.1978, -16.3211) (-5.1959, -16.3153) (-5.1941, -16.3095) (-5.1923, -16.3038) (-5.1905, -16.2981) (-5.1888, -16.2925) (-5.1871, -16.2869) (-5.1854, -16.2815) (-5.1838, -16.276) (-5.1822, -16.2707) (-5.1806, -16.2654) (-5.179, -16.2601) (-5.1775, -16.2549) (-5.176, -16.2498) (-5.1745, -16.2448) (-5.173, -16.2398) (-5.1716, -16.2349) (-5.1702, -16.23) (-5.1689, -16.2252) (-5.1675, -16.2205) (-5.1662, -16.2158) (-5.1649, -16.2112) (-5.1637, -16.2067) (-5.1625, -16.2023) (-5.1613, -16.1979) (-5.1601, -16.1936) (-5.1589, -16.1893) (-5.1578, -16.1852) (-5.1567, -16.1811) (-5.1557, -16.1771) (-5.1546, -16.1731) (-5.1536, -16.1693) (-5.1527, -16.1655) (-5.1517, -16.1617) (-5.1508, -16.1581) (-5.1499, -16.1545) (-5.149, -16.1511) (-5.1481, -16.1477) (-5.1473, -16.1443) (-5.1465, -16.1411) (-5.1458, -16.1379) (-5.145, -16.1349) (-5.1443, -16.1319) (-5.1436, -16.129) (-5.143, -16.1262) (-5.1423, -16.1234) (-5.1417, -16.1208) (-5.1411, -16.1182) (-5.1406, -16.1158) (-5.14, -16.1134) (-5.1395, -16.1111) (-5.139, -16.1089) (-5.1386, -16.1069) (-5.1381, -16.1049) (-5.1377, -16.103) (-5.1374, -16.1012) (-5.137, -16.0995) (-5.1367, -16.0979) (-5.1363, -16.0964) (-5.1361, -16.095) (-5.1358, -16.0937) (-5.1356, -16.0925) (-5.1354, -16.0915) (-5.1352, -16.0905) (-5.135, -16.0896) (-5.1349, -16.0889) (-5.1348, -16.0884) (-5.1347, -16.0881) (-5.1347, -16.0879) (-5.1346, -16.0878) knots -1 -1 -1 -1 -1 -1 -0.99583333 -0.99166667 -0.9875 -0.98333333 -0.97916667 -0.975 -0.97083333 -0.96666667 -0.9625 -0.95833333 -0.95416667 -0.95 -0.94583333 -0.94166667 -0.9375 -0.93333333 -0.92916667 -0.925 -0.92083333 -0.91666667 -0.9125 -0.90833333 -0.90416667 -0.9 -0.89583333 -0.89166667 -0.8875 -0.88333333 -0.87916667 -0.875 -0.87083333 -0.86666667 -0.8625 -0.85833333 -0.85416667 -0.85 -0.84583333 -0.84166667 -0.8375 -0.83333333 -0.82916667 -0.825 -0.82083333 -0.81666667 -0.8125 -0.80833333 -0.80416667 -0.8 -0.79583333 -0.79166667 -0.7875 -0.78333333 -0.77916667 -0.775 -0.77083333 -0.76666667 -0.7625 -0.75833333 -0.75416667 -0.75 -0.74583333 -0.74166667 -0.7375 -0.73333333 -0.72916667 -0.725 -0.72083333 -0.71666667 -0.7125 -0.70833333 -0.70416667 -0.7 -0.69583333 -0.69166667 -0.6875 -0.68333333 -0.67916667 -0.675 -0.67083333 -0.66666667 -0.6625 -0.65833333 -0.65416667 -0.65 -0.64583333 -0.64166667 -0.6375 -0.63333333 -0.62916667 -0.625 -0.62083333 -0.61666667 -0.6125 -0.60833333 -0.60416667 -0.6 -0.59583333 -0.59166667 -0.5875 -0.58333333 -0.57916667 -0.575 -0.57083333 -0.56666667 -0.5625 -0.55833333 -0.55416667 -0.55 -0.54583333 -0.54166667 -0.5375 -0.53333333 -0.52916667 -0.525 -0.52083333 -0.51666667 -0.5125 -0.50833333 -0.50416667 -0.5 -0.49583333 -0.49166667 -0.4875 -0.48333333 -0.47916667 -0.475 -0.47083333 -0.46666667 -0.4625 -0.45833333 -0.45416667 -0.45 -0.44583333 -0.44166667 -0.4375 -0.43333333 -0.42916667 -0.425 -0.42083333 -0.41666667 -0.4125 -0.40833333 -0.40416667 -0.4 -0.39583333 -0.39166667 -0.3875 -0.38333333 -0.37916667 -0.375 -0.37083333 -0.36666667 -0.3625 -0.35833333 -0.35416667 -0.35 -0.34583333 -0.34166667 -0.3375 -0.33333333 -0.32916667 -0.325 -0.32083333 -0.31666667 -0.3125 -0.30833333 -0.30416667 -0.3 -0.29583333 -0.29166667 -0.2875 -0.28333333 -0.27916667 -0.275 -0.27083333 -0.26666667 -0.2625 -0.25833333 -0.25416667 -0.25 -0.24583333 -0.24166667 -0.2375 -0.23333333 -0.22916667 -0.225 -0.22083333 -0.21666667 -0.2125 -0.20833333 -0.20416667 -0.2 -0.19583333 -0.19166667 -0.1875 -0.18333333 -0.17916667 -0.175 -0.17083333 -0.16666667 -0.1625 -0.15833333 -0.15416667 -0.15 -0.14583333 -0.14166667 -0.1375 -0.13333333 -0.12916667 -0.125 -0.12083333 -0.11666667 -0.1125 -0.10833333 -0.10416667 -0.1 -0.09583333 -0.09166667 -0.0875 -0.08333333 -0.07916667 -0.075 -0.07083333 -0.06666667 -0.0625 -0.05833333 -0.05416667 -0.05 -0.04583333 -0.04166667 -0.0375 -0.03333333 -0.02916667 -0.025 -0.02083333 -0.01666667 -0.0125 -0.00833333 -0.00416667 0 0 0 0 0 0
  spline S3 degree 5 poles (15.9204, -14.0997) (15.9199, -14.097) (15.9189, -14.0917) (15.9174, -14.0837) (15.9154, -14.0731) (15.913, -14.0599) (15.9105, -14.0467) (15.908, -14.0335) (15.9055, -14.0204) (15.9029, -14.0073) (15.9004, -13.9943) (15.8979, -13.9812) (15.8953, -13.9682) (15.8927, -13.9553) (15.8902, -13.9424) (15.8876, -13.9295) (15.885, -13.9166) (15.8824, -13.9038) (15.8798, -13.891) (15.8771, -13.8783) (15.8745, -13.8656) (15.8719, -13.8529) (15.8692, -13.8403) (15.8666, -13.8276) (15.8639, -13.8151) (15.8612, -13.8025) (15.8585, -13.79) (15.8558, -13.7776) (15.8531, -13.7651) (15.8504, -13.7528) (15.8477, -13.7404) (15.8449, -13.7281) (15.8422, -13.7158) (15.8394, -13.7035) (15.8367, -13.6913) (15.8339, -13.6792) (15.8311, -13.667) (15.8283, -13.6549) (15.8255, -13.6428) (15.8227, -13.6308) (15.8199, -13.6188) (15.8171, -13.6069) (15.8143, -13.595) (15.8115, -13.5831) (15.8086, -13.5712) (15.8058, -13.5594) (15.8029, -13.5477) (15.8001, -13.5359) (15.7972, -13.5242) (15.7943, -13.5126) (15.7914, -13.501) (15.7886, -13.4894) (15.7857, -13.4778) (15.7828, -13.4663) (15.7798, -13.4549) (15.7769, -13.4435) (15.774, -13.4321) (15.7711, -13.4207) (15.7682, -13.4094) (15.7652, -13.3982) (15.7623, -13.3869) (15.7593, -13.3757) (15.7564, -13.3646) (15.7534, -13.3535) (15.7504, -13.3424) (15.7475, -13.3314) (15.7445, -13.3204) (15.7415, -13.3094) (15.7385, -13.2985) (15.7355, -13.2877) (15.7325, -13.2768) (15.7295, -13.266) (15.7265, -13.2553) (15.7235, -13.2446) (15.7205, -13.2339) (15.7175, -13.2233) (15.7145, -13.2127) (15.7114, -13.2022) (15.7084, -13.1917) (15.7054, -13.1812) (15.7023, -13.1708) (15.6993, -13.1604) (15.6963, -13.1501) (15.6932, -13.1398) (15.6902, -13.1296) (15.6871, -13.1194) (15.6841, -13.1092) (15.681, -13.0991) (15.6779, -13.089) (15.6749, -13.079) (15.6718, -13.069) (15.6688, -13.059) (15.6657, -13.0491) (15.6626, -13.0393) (15.6596, -13.0294) (15.6565, -13.0197) (15.6534, -13.0099) (15.6503, -13.0003) (15.6473, -12.9906) (15.6442, -12.981) (15.6411, -12.9715) (15.638, -12.962) (15.635, -12.9525) (15.6319, -12.9431) (15.6288, -12.9337) (15.6257, -12.9244) (15.6227, -12.9151) (15.6196, -12.9059) (15.6165, -12.8967) (15.6134, -12.8876) (15.6104, -12.8785) (15.6073, -12.8694) (15.6042, -12.8604) (15.6012, -12.8515) (15.5981, -12.8426) (15.595, -12.8337) (15.592, -12.8249) (15.5889, -12.8161) (15.5859, -12.8074) (15.5828, -12.7988) (15.5798, -12.7901) (15.5767, -12.7816) (15.5737, -12.7731) (15.5706, -12.7646) (15.5676, -12.7562) (15.5645, -12.7478) (15.5615, -12.7394) (15.5585, -12.7312) (15.5555, -12.7229) (15.5524, -12.7148) (15.5494, -12.7066) (15.5464, -12.6986) (15.5434, -12.6905) (15.5404, -12.6826) (15.5374, -12.6746) (15.5344, -12.6668) (15.5315, -12.6589) (15.5285, -12.6512) (15.5255, -12.6434) (15.5226, -12.6358) (15.5196, -12.6282) (15.5166, -12.6206) (15.5137, -12.6131) (15.5108, -12.6056) (15.5078, -12.5982) (15.5049, -12.5909) (15.502, -12.5836) (15.4991, -12.5763) (15.4962, -12.5691) (15.4933, -12.562) (15.4905, -12.5549) (15.4876, -12.5479) (15.4848, -12.5409) (15.4819, -12.534) (15.4791, -12.5271) (15.4762, -12.5203) (15.4734, -12.5136) (15.4706, -12.5069) (15.4678, -12.5002) (15.4651, -12.4936) (15.4623, -12.4871) (15.4595, -12.4806) (15.4568, -12.4742) (15.4541, -12.4679) (15.4514, -12.4616) (15.4486, -12.4553) (15.446, -12.4492) (15.4433, -12.443) (15.4406, -12.437) (15.438, -12.431) (15.4353, -12.425) (15.4327, -12.4192) (15.4301, -12.4133) (15.4275, -12.4076) (15.425, -12.4019) (15.4224, -12.3962) (15.4199, -12.3907) (15.4174, -12.3852) (15.4149, -12.3797) (15.4124, -12.3743) (15.4099, -12.369) (15.4075, -12.3637) (15.405, -12.3585) (15.4026, -12.3534) (15.4002, -12.3483) (15.3979, -12.3433) (15.3955, -12.3384) (15.3932, -12.3335) (15.3909, -12.3287) (15.3886, -12.3239) (15.3863, -12.3193) (15.3841, -12.3147) (15.3819, -12.3101) (15.3797, -12.3056) (15.3775, -12.3012) (15.3754, -12.2969) (15.3733, -12.2926) (15.3712, -12.2884) (15.3691, -12.2843) (15.3671, -12.2802) (15.3651, -12.2763) (15.3631, -12.2723) (15.3611, -12.2685) (15.3592, -12.2647) (15.3573, -12.261) (15.3554, -12.2574) (15.3536, -12.2539) (15.3518, -12.2504) (15.35, -12.247) (15.3482, -12.2437) (15.3465, -12.2404) (15.3449, -12.2372) (15.3432, -12.2341) (15.3416, -12.2311) (15.34, -12.2282) (15.3385, -12.2253) (15.337, -12.2225) (15.3355, -12.2198) (15.3341, -12.2172) (15.3327, -12.2147) (15.3313, -12.2122) (15.33, -12.2099) (15.3287, -12.2076) (15.3275, -12.2054) (15.3263, -12.2033) (15.3252, -12.2012) (15.3241, -12.1993) (15.323, -12.1974) (15.322, -12.1956) (15.321, -12.194) (15.3201, -12.1924) (15.3193, -12.1909) (15.3184, -12.1895) (15.3177, -12.1881) (15.3169, -12.1869) (15.3163, -12.1858) (15.3157, -12.1848) (15.3151, -12.1838) (15.3146, -12.183) (15.3142, -12.1822) (15.3138, -12.1816) (15.3135, -12.1812) (15.3133, -12.1809) (15.3132, -12.1807) (15.3132, -12.1806) knots -1 -1 -1 -1 -1 -1 -0.99583333 -0.99166667 -0.9875 -0.98333333 -0.97916667 -0.975 -0.97083333 -0.96666667 -0.9625 -0.95833333 -0.95416667 -0.95 -0.94583333 -0.94166667 -0.9375 -0.93333333 -0.92916667 -0.925 -0.92083333 -0.91666667 -0.9125 -0.90833333 -0.90416667 -0.9 -0.89583333 -0.89166667 -0.8875 -0.88333333 -0.87916667 -0.875 -0.87083333 -0.86666667 -0.8625 -0.85833333 -0.85416667 -0.85 -0.84583333 -0.84166667 -0.8375 -0.83333333 -0.82916667 -0.825 -0.82083333 -0.81666667 -0.8125 -0.80833333 -0.80416667 -0.8 -0.79583333 -0.79166667 -0.7875 -0.78333333 -0.77916667 -0.775 -0.77083333 -0.76666667 -0.7625 -0.75833333 -0.75416667 -0.75 -0.74583333 -0.74166667 -0.7375 -0.73333333 -0.72916667 -0.725 -0.72083333 -0.71666667 -0.7125 -0.70833333 -0.70416667 -0.7 -0.69583333 -0.69166667 -0.6875 -0.68333333 -0.67916667 -0.675 -0.67083333 -0.66666667 -0.6625 -0.65833333 -0.65416667 -0.65 -0.64583333 -0.64166667 -0.6375 -0.63333333 -0.62916667 -0.625 -0.62083333 -0.61666667 -0.6125 -0.60833333 -0.60416667 -0.6 -0.59583333 -0.59166667 -0.5875 -0.58333333 -0.57916667 -0.575 -0.57083333 -0.56666667 -0.5625 -0.55833333 -0.55416667 -0.55 -0.54583333 -0.54166667 -0.5375 -0.53333333 -0.52916667 -0.525 -0.52083333 -0.51666667 -0.5125 -0.50833333 -0.50416667 -0.5 -0.49583333 -0.49166667 -0.4875 -0.48333333 -0.47916667 -0.475 -0.47083333 -0.46666667 -0.4625 -0.45833333 -0.45416667 -0.45 -0.44583333 -0.44166667 -0.4375 -0.43333333 -0.42916667 -0.425 -0.42083333 -0.41666667 -0.4125 -0.40833333 -0.40416667 -0.4 -0.39583333 -0.39166667 -0.3875 -0.38333333 -0.37916667 -0.375 -0.37083333 -0.36666667 -0.3625 -0.35833333 -0.35416667 -0.35 -0.34583333 -0.34166667 -0.3375 -0.33333333 -0.32916667 -0.325 -0.32083333 -0.31666667 -0.3125 -0.30833333 -0.30416667 -0.3 -0.29583333 -0.29166667 -0.2875 -0.28333333 -0.27916667 -0.275 -0.27083333 -0.26666667 -0.2625 -0.25833333 -0.25416667 -0.25 -0.24583333 -0.24166667 -0.2375 -0.23333333 -0.22916667 -0.225 -0.22083333 -0.21666667 -0.2125 -0.20833333 -0.20416667 -0.2 -0.19583333 -0.19166667 -0.1875 -0.18333333 -0.17916667 -0.175 -0.17083333 -0.16666667 -0.1625 -0.15833333 -0.15416667 -0.15 -0.14583333 -0.14166667 -0.1375 -0.13333333 -0.12916667 -0.125 -0.12083333 -0.11666667 -0.1125 -0.10833333 -0.10416667 -0.1 -0.09583333 -0.09166667 -0.0875 -0.08333333 -0.07916667 -0.075 -0.07083333 -0.06666667 -0.0625 -0.05833333 -0.05416667 -0.05 -0.04583333 -0.04166667 -0.0375 -0.03333333 -0.02916667 -0.025 -0.02083333 -0.01666667 -0.0125 -0.00833333 -0.00416667 0 0 0 0 0 0
  arc A14 (27.0873, 27.5758) -> (26.5997, 28.4204) centre (0, 12.5) ccw
  arc A15 (24.4297, 27.6575) -> (23.7836, 28.6526) centre (0, 12.5) ccw
  line L23 (24.0271, 28.818) -> (24.0278, 28.8184)
  arc A16 (25.8803, 25.0209) -> (25.3417, 26.078) centre (0, 12.5) ccw